Autodesk Fusion 360 part; units mm, degrees
(part 3 of 13)
  line L1812 (141.624, -72.5436) -> (141.627, -72.5391)
  line L1813 (141.22, -72.9625) -> (141.287, -72.9157)
  line L1814 (144.496, -71.2807) -> (144.455, -71.3702)
  line L1815 (141.745, -81.2151) -> (141.668, -81.0591)
  line L1816 (100.087, -70.3919) -> (100.08, -70.4118)
  line L1817 (99.926, -70.1408) -> (99.9333, -70.1465)
  line L1818 (100.059, -70.284) -> (100.065, -70.3008)
  line L1819 (99.9486, -70.1553) -> (99.9571, -70.1588)
  line L1820 (100.08, -70.3362) -> (100.087, -70.3561)
  line L1821 (88.7182, -70.3919) -> (88.7208, -70.374)
  line L1822 (99.8082, -70.6072) -> (99.801, -70.6015)
  line L1823 (99.9871, -70.1888) -> (100.059, -70.284)
  line L1824 (88.8796, -70.1408) -> (88.9008, -70.1378)
  line L1825 (99.9049, -70.6102) -> (99.8851, -70.6182)
  line L1826 (88.8571, -70.5927) -> (88.8485, -70.5892)
  line L1827 (100.085, -70.374) -> (100.087, -70.3919)
  line L1828 (88.8185, -70.1888) -> (88.8353, -70.1756)
  line L1829 (100.087, -70.3561) -> (100.085, -70.374)
  line L1830 (99.9871, -70.5592) -> (99.9703, -70.5724)
  line L1831 (88.7404, -70.4472) -> (88.7292, -70.4329)
  line L1832 (88.9474, -70.6169) -> (88.9385, -70.6192)
  line L1833 (88.9008, -70.6102) -> (88.8796, -70.6072)
  line L1834 (99.8851, -70.6182) -> (99.876, -70.6169)
  line L1835 (88.9297, -70.1311) -> (88.9385, -70.1288)
  line L1836 (100.059, -70.464) -> (99.9871, -70.5592)
  line L1837 (99.9571, -70.1588) -> (99.9703, -70.1756)
  line L1838 (88.7471, -70.464) -> (88.7404, -70.4472)
  line L1839 (88.9206, -70.6182) -> (88.9008, -70.6102)
  line L1840 (100.065, -70.4472) -> (100.059, -70.464)
  line L1841 (88.8353, -70.5724) -> (88.8185, -70.5592)
  line L1842 (88.8485, -70.5892) -> (88.8353, -70.5724)
  line L1843 (99.9703, -70.5724) -> (99.9571, -70.5892)
  line L1844 (88.8635, -70.1489) -> (88.8724, -70.1465)
  line L1845 (88.8796, -70.6072) -> (88.8724, -70.6015)
  line L1846 (99.9571, -70.5892) -> (99.9486, -70.5927)
  line L1847 (99.9049, -70.1378) -> (99.926, -70.1408)
  line L1848 (99.9421, -70.1489) -> (99.9486, -70.1553)
  line L1849 (100.08, -70.4118) -> (100.076, -70.4329)
  line L1850 (99.9333, -70.1465) -> (99.9421, -70.1489)
  line L1851 (88.9385, -70.1288) -> (88.9474, -70.1311)
  line L1852 (99.926, -70.6072) -> (99.9049, -70.6102)
  line L1853 (99.7921, -70.5991) -> (99.7856, -70.5927)
  line L1854 (88.8635, -70.5991) -> (88.8571, -70.5927)
  line L1855 (99.9486, -70.5927) -> (99.9421, -70.5991)
  line L1856 (99.8583, -70.6169) -> (99.8492, -70.6182)
  line L1857 (88.9297, -70.6169) -> (88.9206, -70.6182)
  line L1858 (88.7471, -70.284) -> (88.8185, -70.1888)
  line L1859 (99.6547, -70.3362) -> (99.6577, -70.3151)
  line L1860 (100.065, -70.3008) -> (100.076, -70.3151)
  line L1861 (99.9703, -70.1756) -> (99.9871, -70.1888)
  line L1862 (88.9385, -70.6192) -> (88.9297, -70.6169)
  line L1863 (88.8571, -70.1553) -> (88.8635, -70.1489)
  line L1864 (88.8353, -70.1756) -> (88.8485, -70.1588)
  line L1865 (88.8485, -70.1588) -> (88.8571, -70.1553)
  line L1866 (99.9421, -70.5991) -> (99.9333, -70.6015)
  line L1867 (88.9206, -70.1298) -> (88.9297, -70.1311)
  line L1868 (88.7404, -70.3008) -> (88.7471, -70.284)
  line L1869 (88.8724, -70.1465) -> (88.8796, -70.1408)
  line L1870 (88.7261, -70.3362) -> (88.7292, -70.3151)
  line L1871 (100.076, -70.3151) -> (100.08, -70.3362)
  line L1872 (88.7292, -70.3151) -> (88.7404, -70.3008)
  line L1873 (88.9008, -70.1378) -> (88.9206, -70.1298)
  line L1874 (99.8851, -70.1298) -> (99.9049, -70.1378)
  line L1875 (88.8724, -70.6015) -> (88.8635, -70.5991)
  line L1876 (99.9333, -70.6015) -> (99.926, -70.6072)
  line L1877 (100.076, -70.4329) -> (100.065, -70.4472)
  line L1878 (99.876, -70.1311) -> (99.8851, -70.1298)
  line L1879 (147.689, -96.129) -> (147.754, -96.0856)
  line L1880 (99.7771, -70.5892) -> (99.7639, -70.5724)
  line L1881 (99.6493, -70.374) -> (99.6468, -70.3561)
  line L1882 (99.6757, -70.284) -> (99.7471, -70.1888)
  line L1883 (99.7639, -70.5724) -> (99.7471, -70.5592)
  line L1884 (147.53, -95.6243) -> (147.397, -95.7052)
  line L1885 (99.8082, -70.1408) -> (99.8293, -70.1378)
  line L1886 (146.874, -95.6199) -> (146.867, -95.6177)
  line L1887 (99.7856, -70.1553) -> (99.7921, -70.1489)
  line L1888 (147.754, -96.0856) -> (147.776, -96.0811)
  line L1889 (99.8492, -70.6182) -> (99.8293, -70.6102)
  line L1890 (147.77, -95.5641) -> (147.766, -95.5631)
  line L1891 (147.689, -96.9618) -> (147.645, -96.8969)
  line L1892 (146.8, -95.5969) -> (146.71, -95.5686)
  line L1893 (99.6468, -70.3919) -> (99.6493, -70.374)
  line L1894 (99.8671, -70.1288) -> (99.876, -70.1311)
  line L1895 (147.772, -95.5653) -> (147.77, -95.5641)
  line L1896 (99.7471, -70.5592) -> (99.6757, -70.464)
  line L1897 (147.544, -95.6181) -> (147.53, -95.6243)
  line L1898 (99.7639, -70.1756) -> (99.7771, -70.1588)
  line L1899 (99.7771, -70.1588) -> (99.7856, -70.1553)
  line L1900 (99.8293, -70.1378) -> (99.8492, -70.1298)
  line L1901 (147.645, -96.1939) -> (147.689, -96.129)
  line L1902 (147.63, -96.2704) -> (147.645, -96.1939)
  line L1903 (146.867, -95.6177) -> (146.8, -95.5969)
  line L1904 (147.021, -95.7088) -> (146.874, -95.6199)
  line L1905 (147.385, -95.7145) -> (147.295, -95.8046)
  line L1906 (144.778, -95.5619) -> (144.522, -95.5619)
  line L1907 (99.6757, -70.464) -> (99.6689, -70.4472)
  line L1908 (99.6468, -70.3561) -> (99.6547, -70.3362)
  line L1909 (146.867, -95.6177) -> (146.867, -95.6177)
  line L1910 (147.295, -95.8046) -> (147.232, -95.8387)
  line L1911 (99.8293, -70.6102) -> (99.8082, -70.6072)
  line L1912 (99.7471, -70.1888) -> (99.7639, -70.1756)
  line L1913 (99.6689, -70.3008) -> (99.6757, -70.284)
  line L1914 (99.8671, -70.6192) -> (99.8583, -70.6169)
  line L1915 (99.6689, -70.4472) -> (99.6577, -70.4329)
  line L1916 (147.397, -95.7052) -> (147.385, -95.7145)
  line L1917 (99.801, -70.1465) -> (99.8082, -70.1408)
  line L1918 (99.7921, -70.1489) -> (99.801, -70.1465)
  line L1919 (146.637, -95.5619) -> (146.634, -95.5619)
  line L1920 (99.801, -70.6015) -> (99.7921, -70.5991)
  line L1921 (147.707, -95.5685) -> (147.694, -95.5711)
  line L1922 (99.8583, -70.1311) -> (99.8671, -70.1288)
  line L1923 (147.776, -96.0811) -> (147.776, -95.5805)
  line L1924 (147.754, -97.0052) -> (147.689, -96.9618)
  line L1925 (147.645, -96.8969) -> (147.63, -96.8204)
  line L1926 (99.876, -70.6169) -> (99.8671, -70.6192)
  line L1927 (147.776, -95.5805) -> (147.772, -95.5653)
  line L1928 (147.232, -95.8387) -> (147.162, -95.8336)
  line L1929 (99.8492, -70.1298) -> (99.8583, -70.1311)
  line L1930 (99.6577, -70.3151) -> (99.6689, -70.3008)
  line L1931 (147.116, -95.8046) -> (147.021, -95.7088)
  line L1932 (147.63, -96.8204) -> (147.63, -96.2704)
  line L1933 (147.162, -95.8336) -> (147.116, -95.8046)
  line L1934 (145.036, -95.5619) -> (145.033, -95.5619)
  line L1935 (144.522, -95.5619) -> (144.52, -95.5622)
  line L1936 (99.6577, -70.4329) -> (99.6547, -70.4118)
  line L1937 (147.694, -95.5711) -> (147.544, -95.6181)
  line L1938 (147.766, -95.5631) -> (147.707, -95.5685)
  line L1939 (146.71, -95.5686) -> (146.637, -95.5619)
  line L1940 (145.033, -95.5619) -> (144.778, -95.5619)
  line L1941 (99.7856, -70.5927) -> (99.7771, -70.5892)
  line L1942 (99.6547, -70.4118) -> (99.6468, -70.3919)
  line L1943 (145.265, -95.6177) -> (145.265, -95.6177)
  line L1944 (145.199, -95.5969) -> (145.109, -95.5686)
  line L1945 (146.121, -95.5622) -> (146.121, -95.5622)
  line L1946 (143.762, -93.8918) -> (143.762, -93.8639)
  line L1947 (145.74, -95.7088) -> (145.669, -95.7799)
  line L1948 (145.606, -95.8139) -> (145.536, -95.8088)
  line L1949 (145.887, -95.6199) -> (145.74, -95.7088)
  line L1950 (143.762, -93.9826) -> (143.763, -93.9714)
  line L1951 (143.745, -93.7376) -> (143.745, -93.7376)
  line L1952 (144.293, -95.6177) -> (144.285, -95.6199)
  line L1953 (143.762, -93.86) -> (143.761, -93.8481)
  line L1954 (143.981, -95.8383) -> (143.91, -95.8332)
  line L1955 (145.894, -95.6177) -> (145.894, -95.6177)
  line L1956 (146.044, -95.5706) -> (146.044, -95.5706)
  line L1957 (145.536, -95.8088) -> (145.491, -95.7799)
  line L1958 (146.124, -95.5619) -> (146.121, -95.5622)
  line L1959 (143.762, -93.8639) -> (143.762, -93.86)
  line L1960 (144.519, -95.5622) -> (144.486, -95.5653)
  line L1961 (143.75, -93.7638) -> (143.747, -93.745)
  line L1962 (143.757, -93.795) -> (143.754, -93.7845)
  line L1963 (143.91, -95.8332) -> (143.865, -95.8043)
  line L1964 (145.109, -95.5686) -> (145.036, -95.5619)
  line L1965 (143.76, -93.8118) -> (143.76, -93.8039)
  line L1966 (143.765, -95.6765) -> (143.762, -95.6497)
  line L1967 (143.763, -93.9714) -> (143.765, -93.9639)
  line L1968 (146.044, -95.5706) -> (145.894, -95.6177)
  line L1969 (145.419, -95.7088) -> (145.273, -95.6199)
  line L1970 (146.05, -95.5686) -> (146.044, -95.5706)
  line L1971 (143.747, -93.745) -> (143.745, -93.7376)
  line L1972 (146.087, -95.5653) -> (146.05, -95.5686)
  line L1973 (145.894, -95.6177) -> (145.887, -95.6199)
  line L1974 (145.265, -95.6177) -> (145.199, -95.5969)
  line L1975 (146.121, -95.5622) -> (146.087, -95.5653)
  line L1976 (145.491, -95.7799) -> (145.419, -95.7088)
  line L1977 (144.139, -95.7088) -> (144.043, -95.8043)
  line L1978 (144.043, -95.8043) -> (143.981, -95.8383)
  line L1979 (143.745, -93.7376) -> (143.731, -93.7039)
  line L1980 (143.765, -93.9639) -> (143.763, -93.8958)
  line L1981 (143.76, -93.8039) -> (143.757, -93.795)
  line L1982 (143.799, -95.7388) -> (143.765, -95.6765)
  line L1983 (143.762, -95.6497) -> (143.762, -93.9826)
  line L1984 (143.717, -93.6578) -> (143.717, -93.6578)
  line L1985 (145.273, -95.6199) -> (145.265, -95.6177)
  line L1986 (144.486, -95.5653) -> (144.449, -95.5686)
  line L1987 (146.38, -95.5619) -> (146.124, -95.5619)
  line L1988 (144.52, -95.5622) -> (144.519, -95.5622)
  line L1989 (143.763, -93.8958) -> (143.762, -93.8918)
  line L1990 (143.75, -93.7651) -> (143.75, -93.7638)
  line L1991 (144.443, -95.5706) -> (144.293, -95.6177)
  line L1992 (143.865, -95.8043) -> (143.799, -95.7388)
  line L1993 (143.727, -93.6927) -> (143.717, -93.6578)
  line L1994 (143.754, -93.7845) -> (143.75, -93.7651)
  line L1995 (144.449, -95.5686) -> (144.443, -95.5706)
  line L1996 (145.669, -95.7799) -> (145.606, -95.8139)
  line L1997 (146.634, -95.5619) -> (146.38, -95.5619)
  line L1998 (144.285, -95.6199) -> (144.139, -95.7088)
  line L1999 (144.443, -95.5706) -> (144.443, -95.5706)
  line L2000 (143.731, -93.7039) -> (143.727, -93.6927)
  line L2001 (145.48, -82.2318) -> (145.48, -82.2318)
  line L2002 (143.634, -93.5124) -> (143.619, -93.4981)
  line L2003 (145.955, -82.3539) -> (145.955, -82.3539)
  line L2004 (143.638, -93.5193) -> (143.634, -93.5124)
  line L2005 (145.963, -82.3547) -> (145.963, -82.3547)
  line L2006 (146.164, -82.3559) -> (146.166, -82.3557)
  line L2007 (146.346, -82.3413) -> (146.351, -82.3409)
  line L2008 (145.988, -82.3558) -> (145.989, -82.3559)
  line L2009 (145.815, -82.3297) -> (145.955, -82.3539)
  line L2010 (143.588, -93.4616) -> (143.56, -93.4385)
  line L2011 (144.293, -95.6177) -> (144.293, -95.6177)
  line L2012 (142.604, -92.4116) -> (142.615, -92.3365)
  line L2013 (145.059, -81.9624) -> (145.059, -81.9624)
  line L2014 (143.717, -93.6578) -> (143.715, -93.6502)
  line L2015 (146.166, -82.3557) -> (146.346, -82.3413)
  line L2016 (145.48, -82.2318) -> (145.705, -82.3096)
  line L2017 (143.552, -93.4305) -> (142.987, -92.8662)
  line L2018 (142.617, -92.2782) -> (142.604, -92.136)
  line L2019 (143.656, -93.5505) -> (143.638, -93.5193)
  line L2020 (143.715, -93.6502) -> (143.705, -93.6328)
  line L2021 (143.689, -93.5962) -> (143.663, -93.5604)
  line L2022 (143.761, -93.8481) -> (143.76, -93.8118)
  line L2023 (142.606, -92.4564) -> (142.604, -92.4116)
  line L2024 (143.594, -93.4667) -> (143.588, -93.4616)
  line L2025 (142.987, -92.8662) -> (142.64, -92.5187)
  line L2026 (142.599, -92.0811) -> (142.599, -92.0811)
  line L2027 (143.663, -93.5604) -> (143.656, -93.5505)
  line L2028 (145.258, -82.1141) -> (145.258, -82.1141)
  line L2029 (145.059, -81.9624) -> (145.25, -82.1086)
  line L2030 (145.705, -82.3096) -> (145.712, -82.3118)
  line L2031 (143.599, -93.4731) -> (143.594, -93.4667)
  line L2032 (143.56, -93.4385) -> (143.552, -93.4305)
  line L2033 (145.285, -82.1286) -> (145.475, -82.2302)
  line L2034 (145.989, -82.3559) -> (146.164, -82.3559)
  line L2035 (145.25, -82.1086) -> (145.254, -82.1117)
  line L2036 (145.475, -82.2302) -> (145.48, -82.2318)
  line L2037 (145.959, -82.3545) -> (145.963, -82.3547)
  line L2038 (142.604, -92.136) -> (142.599, -92.0811)
  line L2039 (142.64, -92.5187) -> (142.606, -92.4564)
  line L2040 (143.619, -93.4981) -> (143.606, -93.4831)
  line L2041 (143.588, -93.4616) -> (143.588, -93.4616)
  line L2042 (143.705, -93.6328) -> (143.696, -93.615)
  line L2043 (146.166, -82.3557) -> (146.166, -82.3557)
  line L2044 (145.258, -82.1141) -> (145.285, -82.1286)
  line L2045 (146.589, -82.2822) -> (146.594, -82.281)
  line L2046 (143.696, -93.615) -> (143.691, -93.6036)
  line L2047 (142.615, -92.3365) -> (142.617, -92.2782)
  line L2048 (146.356, -82.3397) -> (146.589, -82.2822)
  line L2049 (143.606, -93.4831) -> (143.599, -93.4731)
  line L2050 (145.712, -82.3118) -> (145.815, -82.3297)
  line L2051 (145.055, -81.9594) -> (145.059, -81.9624)
  line L2052 (143.691, -93.6036) -> (143.689, -93.5962)
  line L2053 (146.356, -82.3397) -> (146.356, -82.3397)
  line L2054 (147.385, -81.6898) -> (147.511, -81.473)
  line L2055 (147.663, -80.7428) -> (147.635, -80.4937)
  line L2056 (146.494, -79.2846) -> (146.49, -79.283)
  line L2057 (146.246, -72.9976) -> (146.28, -72.9625)
  line L2058 (145.25, -82.1086) -> (145.25, -82.1086)
  line L2059 (147.457, -80.0209) -> (147.333, -79.8377)
  line L2060 (147.511, -81.473) -> (147.526, -81.4327)
  line L2061 (147.226, -81.8835) -> (147.385, -81.6898)
  line L2062 (145.254, -82.1117) -> (145.258, -82.1141)
  line L2063 (147.625, -80.4586) -> (147.568, -80.2573)
  line L2064 (147.651, -80.9983) -> (147.652, -80.9934)
  line L2065 (146.821, -82.185) -> (146.825, -82.183)
  line L2066 (147.462, -80.0297) -> (147.462, -80.0297)
  line L2067 (146.687, -72.5391) -> (146.689, -72.5341)
  line L2068 (146.347, -72.9157) -> (146.4, -72.8783)
  line L2069 (147.322, -79.8218) -> (147.322, -79.8218)
  line L2070 (147.635, -80.4937) -> (147.625, -80.4586)
  line L2071 (147.566, -80.2524) -> (147.564, -80.2478)
  line L2072 (146.594, -82.281) -> (146.599, -82.2791)
  line L2073 (145.955, -82.3539) -> (145.959, -82.3545)
  line L2074 (146.821, -82.185) -> (146.821, -82.185)
  line L2075 (147.652, -80.9934) -> (147.657, -80.8824)
  line L2076 (147.599, -81.2436) -> (147.601, -81.2389)
  line L2077 (147.564, -80.2478) -> (147.564, -80.2478)
  line L2078 (147.462, -80.0297) -> (147.46, -80.0251)
  line L2079 (147.601, -81.2389) -> (147.607, -81.2096)
  line L2080 (147.657, -80.8824) -> (147.663, -80.7428)
  line L2081 (146.599, -82.2791) -> (146.599, -82.2791)
  line L2082 (147.037, -82.0494) -> (147.226, -81.8835)
  line L2083 (146.346, -82.3413) -> (146.346, -82.3413)
  line L2084 (145.963, -82.3547) -> (145.988, -82.3558)
  line L2085 (147.333, -79.8377) -> (147.322, -79.8218)
  line L2086 (146.599, -82.2791) -> (146.821, -82.185)
  line L2087 (145.988, -82.3558) -> (145.988, -82.3558)
  line L2088 (147.526, -81.4327) -> (147.599, -81.2436)
  line L2089 (147.568, -80.2572) -> (147.566, -80.2524)
  line L2090 (147.568, -80.2573) -> (147.568, -80.2572)
  line L2091 (147.46, -80.0251) -> (147.457, -80.0209)
  line L2092 (147.322, -79.8218) -> (147.319, -79.8177)
  line L2093 (146.825, -82.183) -> (147.037, -82.0494)
  line L2094 (146.4, -72.8783) -> (146.405, -72.8751)
  line L2095 (147.564, -80.2478) -> (147.462, -80.0297)
  line L2096 (147.607, -81.2096) -> (147.651, -80.9983)
  line L2097 (146.4, -72.8783) -> (146.4, -72.8783)
  line L2098 (147.319, -79.8177) -> (147.147, -79.6354)
  line L2099 (146.351, -82.3409) -> (146.356, -82.3397)
  line L2100 (146.405, -72.8751) -> (146.561, -72.7194)
  line L2101 (146.684, -72.5436) -> (146.687, -72.5391)
  line L2102 (146.905, -79.4602) -> (146.731, -79.367)
  line L2103 (146.561, -72.7194) -> (146.59, -72.6768)
  line L2104 (147.111, -79.6076) -> (146.952, -79.4862)
  line L2105 (146.226, -73.0658) -> (146.246, -72.9976)
  line L2106 (146.331, -79.2555) -> (146.267, -79.2242)
  line L2107 (146.485, -79.2821) -> (146.485, -79.2821)
  line L2108 (146.952, -79.4862) -> (146.952, -79.4862)
  line L2109 (146.59, -72.6768) -> (146.684, -72.5436)
  line L2110 (146.684, -72.5436) -> (146.684, -72.5436)
  line L2111 (146.689, -72.5341) -> (146.689, -72.5341)
  line L2112 (146.727, -79.3646) -> (146.722, -79.363)
  line L2113 (146.28, -72.9625) -> (146.347, -72.9157)
  line L2114 (146.722, -79.363) -> (146.494, -79.2846)
  line L2115 (146.722, -79.363) -> (146.722, -79.363)
  line L2116 (146.267, -79.2242) -> (146.23, -79.1634)
  line L2117 (146.226, -79.1314) -> (146.226, -73.0658)
  line L2118 (147.147, -79.6354) -> (147.111, -79.6076)
  line L2119 (146.731, -79.367) -> (146.727, -79.3646)
  line L2120 (146.948, -79.4831) -> (146.905, -79.4602)
  line L2121 (146.49, -79.283) -> (146.485, -79.2821)
  line L2122 (146.952, -79.4862) -> (146.948, -79.4831)
  line L2123 (146.23, -79.1634) -> (146.226, -79.1314)
  line L2124 (146.778, -72.3445) -> (146.78, -72.3395)
  line L2125 (146.689, -72.5341) -> (146.778, -72.3445)
  line L2126 (145.593, -70.6441) -> (145.373, -70.6633)
  line L2127 (146.561, -71.0954) -> (146.405, -70.9397)
  line L2128 (146.687, -71.2757) -> (146.658, -71.2339)
  line L2129 (146.689, -71.2807) -> (146.689, -71.2807)
  line L2130 (146.837, -71.688) -> (146.78, -71.4753)
  line L2131 (145.161, -70.7203) -> (145.067, -70.7638)
  line L2132 (145.067, -70.7638) -> (144.966, -70.811)
  line L2133 (146.856, -71.9074) -> (146.837, -71.688)
  line L2134 (145.373, -70.6633) -> (145.161, -70.7203)
  line L2135 (144.785, -70.9365) -> (144.781, -70.9397)
  line L2136 (144.781, -70.9397) -> (144.625, -71.0954)
  line L2137 (145.812, -70.6633) -> (145.593, -70.6441)
  line L2138 (144.961, -70.8133) -> (144.957, -70.8165)
  line L2139 (146.564, -71.0999) -> (146.561, -71.0954)
  line L2140 (146.405, -70.9397) -> (146.224, -70.8133)
  line L2141 (144.957, -70.8165) -> (144.785, -70.9365)
  line L2142 (144.957, -70.8165) -> (144.957, -70.8165)
  line L2143 (144.625, -71.0954) -> (144.622, -71.0999)
  line L2144 (146.689, -71.2807) -> (146.687, -71.2757)
  line L2145 (146.658, -71.2339) -> (146.564, -71.0999)
  line L2146 (146.837, -72.1268) -> (146.856, -71.9074)
  line L2147 (144.966, -70.811) -> (144.966, -70.811)
  line L2148 (146.731, -71.3702) -> (146.689, -71.2807)
  line L2149 (146.78, -72.3395) -> (146.837, -72.1268)
  line L2150 (146.564, -71.0999) -> (146.564, -71.0999)
  line L2151 (144.966, -70.811) -> (144.961, -70.8133)
  line L2152 (144.785, -70.9365) -> (144.785, -70.9365)
  line L2153 (144.785, -72.8783) -> (144.839, -72.9157)
  line L2154 (146.224, -70.8133) -> (146.025, -70.7203)
  line L2155 (144.785, -72.8783) -> (144.785, -72.8783)
  line L2156 (146.78, -71.4753) -> (146.731, -71.3702)
  line L2157 (146.025, -70.7203) -> (145.812, -70.6633)
  line L2158 (144.595, -72.6768) -> (144.625, -72.7194)
  line L2159 (146.485, -79.2821) -> (146.331, -79.2555)
  line L2160 (149.909, -80.5669) -> (149.743, -80.582)
  line L2161 (148.697, -80.5093) -> (148.707, -80.5177)
  line L2162 (150.385, -80.9281) -> (150.394, -80.9227)
  line L2163 (150.436, -80.8938) -> (150.444, -80.8833)
  line L2164 (149.764, -81.0945) -> (149.972, -81.0763)
  line L2165 (149.08, -80.1512) -> (149.078, -80.1468)
  line L2166 (149.082, -80.8944) -> (149.122, -80.9227)
  line L2167 (149.753, -81.0945) -> (149.764, -81.0945)
  line L2168 (148.668, -80.4681) -> (148.697, -80.5093)
  line L2169 (150.077, -80.51) -> (150.068, -80.5152)
  line L2170 (150.394, -80.9227) -> (150.436, -80.8938)
  line L2171 (149.079, -80.8706) -> (149.073, -80.8824)
  line L2172 (149.073, -80.8824) -> (149.082, -80.8944)
  line L2173 (148.57, -80.2588) -> (148.574, -80.2691)
  line L2174 (149.332, -81.0203) -> (149.534, -81.0744)
  line L2175 (149.534, -81.0744) -> (149.545, -81.0763)
  line L2176 (150.068, -80.5152) -> (149.909, -80.5669)
  line L2177 (148.516, -80.0568) -> (148.57, -80.2588)
  line L2178 (148.721, -80.5107) -> (149.08, -80.1512)
  line L2179 (150.437, -80.8699) -> (150.077, -80.51)
  line L2180 (148.662, -80.4586) -> (148.668, -80.4681)
  line L2181 (149.972, -81.0763) -> (149.983, -81.0744)
  line L2182 (150.185, -81.0203) -> (150.195, -81.0165)
  line L2183 (150.444, -80.8833) -> (150.437, -80.8699)
  line L2184 (150.195, -81.0165) -> (150.385, -80.9281)
  line L2185 (149.577, -80.5599) -> (149.441, -80.5092)
  circle A0 centre (105.131, -90.8304) radius 0.2
  circle A1 centre (95.4532, -98.5774) radius 0.2
  circle A2 centre (149.733, -79.8322) radius 0.2
  line L2186 (149.764, -78.5699) -> (149.753, -78.5699)
  line L2187 (149.545, -78.5881) -> (149.534, -78.59)
  circle A3 centre (100.914, -89.8144) radius 0.2
  line L2188 (149.534, -78.59) -> (149.332, -78.6441)
  circle A4 centre (124.028, -105.486) radius 0.2
  line L2189 (149.073, -78.7811) -> (149.08, -78.7945)
  circle A5 centre (91.2368, -97.3582) radius 0.2
  line L2190 (149.753, -78.5699) -> (149.545, -78.5881)
  circle A6 centre (96.8756, -86.4362) radius 0.2
  circle A7 centre (107.061, -117.678) radius 0.2
  circle A8 centre (118.694, -110.109) radius 0.2
  line L2191 (149.08, -78.7945) -> (149.439, -79.1536)
  line L2192 (149.081, -78.7706) -> (149.073, -78.7811)
  circle A9 centre (146.444, -102.87) radius 0.2
  line L2193 (149.332, -78.6441) -> (149.322, -78.6479)
  circle A10 centre (102.87, -116.281) radius 0.2
  circle A11 centre (91.3739, -95.631) radius 0.2
  circle A12 centre (105.867, -119.151) radius 0.2
  circle A13 centre (91.1352, -91.8464) radius 0.2
  line L2194 (149.122, -78.7417) -> (149.081, -78.7706)
  circle A14 centre (127.82, -93.8319) radius 0.2
  circle A15 centre (91.2368, -94.4372) radius 0.2
  line L2195 (148.496, -79.8377) -> (148.514, -80.046)
  line L2196 (150.435, -78.77) -> (150.394, -78.7417)
  line L2197 (149.93, -79.102) -> (150.077, -79.1545)
  line L2198 (148.516, -79.6076) -> (148.514, -79.6184)
  line L2199 (148.514, -79.6184) -> (148.496, -79.8267)
  circle A16 centre (86.9442, -111.658) radius 0.2
  line L2200 (149.322, -78.6479) -> (149.132, -78.7363)
  line L2201 (150.385, -78.7363) -> (150.195, -78.6479)
  line L2202 (148.708, -79.1466) -> (148.696, -79.1559)
  circle A17 centre (86.8426, -104.191) radius 0.2
  line L2203 (149.132, -78.7363) -> (149.122, -78.7417)
  line L2204 (148.514, -80.046) -> (148.516, -80.0568)
  line L2205 (149.078, -80.1468) -> (149.025, -79.9881)
  line L2206 (148.662, -79.2058) -> (148.574, -79.3953)
  line L2207 (149.012, -101.459) -> (149.012, -101.459)
  line L2208 (149.368, -101.344) -> (149.361, -101.346)
  line L2209 (149.659, -101.366) -> (149.565, -101.346)
  line L2210 (149.363, -98.3228) -> (149.37, -98.3327)
  line L2211 (149.385, -98.3579) -> (149.392, -98.3708)
  line L2212 (149.432, -98.4165) -> (149.438, -98.4216)
  line L2213 (149.311, -98.233) -> (149.315, -98.2398)
  line L2214 (149.466, -98.4447) -> (149.474, -98.4527)
  line L2215 (149.811, -98.8412) -> (149.811, -101.242)
  line L2216 (148.634, -101.873) -> (148.629, -101.881)
  line L2217 (149.006, -101.462) -> (148.852, -101.574)
  line L2218 (149.308, -101.357) -> (149.181, -101.384)
  line L2219 (149.342, -98.2934) -> (149.363, -98.3228)
  line L2220 (149.281, -98.1456) -> (149.295, -98.1793)
  line L2221 (149.37, -98.3327) -> (149.385, -98.3579)
  line L2222 (149.808, -98.8144) -> (149.811, -98.8412)
  line L2223 (149.181, -101.384) -> (149.175, -101.387)
  line L2224 (149.277, -98.1275) -> (149.279, -98.1382)
  line L2225 (149.392, -98.3708) -> (149.407, -98.3851)
  line L2226 (149.272, -98.0987) -> (149.276, -98.1181)
  line L2227 (149.276, -98.1181) -> (149.277, -98.1275)
  line L2228 (148.852, -101.574) -> (148.724, -101.716)
  line L2229 (149.175, -101.387) -> (149.012, -101.459)
  line L2230 (149.012, -101.459) -> (149.006, -101.462)
  line L2231 (148.337, -102.284) -> (148.32, -102.261)
  line L2232 (149.281, -98.1456) -> (149.281, -98.1456)
  line L2233 (149.565, -101.346) -> (149.565, -101.346)
  line L2234 (148.57, -102.063) -> (148.569, -102.07)
  line L2235 (149.407, -98.3851) -> (149.42, -98.4001)
  line L2236 (148.288, -102.206) -> (148.16, -102.064)
  line L2237 (149.42, -98.4001) -> (149.432, -98.4165)
  line L2238 (149.361, -101.346) -> (149.361, -101.346)
  line L2239 (148.569, -102.07) -> (148.569, -102.07)
  line L2240 (149.474, -98.4527) -> (149.774, -98.7521)
  line L2241 (149.337, -98.287) -> (149.342, -98.2934)
  line L2242 (148.569, -102.07) -> (148.554, -102.212)
  line L2243 (149.342, -98.2934) -> (149.342, -98.2934)
  line L2244 (149.811, -101.242) -> (149.791, -101.311)
  line L2245 (148.16, -102.064) -> (148.061, -101.992)
  line L2246 (149.33, -98.2682) -> (149.337, -98.287)
  line L2247 (149.438, -98.4216) -> (149.466, -98.4447)
  line L2248 (149.737, -101.357) -> (149.667, -101.367)
  line L2249 (149.361, -101.346) -> (149.308, -101.357)
  line L2250 (148.629, -101.881) -> (148.57, -102.063)
  line L2251 (148.724, -101.716) -> (148.721, -101.722)
  line L2252 (148.32, -102.261) -> (148.288, -102.206)
  line L2253 (149.774, -98.7521) -> (149.808, -98.8144)
  line L2254 (148.398, -102.32) -> (148.337, -102.284)
  line L2255 (147.837, -101.877) -> (147.831, -101.874)
  line L2256 (148.469, -102.318) -> (148.398, -102.32)
  line L2257 (148.721, -101.722) -> (148.634, -101.873)
  line L2258 (148.554, -102.212) -> (148.527, -102.277)
  line L2259 (149.667, -101.367) -> (149.659, -101.366)
  line L2260 (149.565, -101.346) -> (149.559, -101.344)
  line L2261 (147.26, -101.877) -> (147.26, -101.877)
  line L2262 (148.527, -102.277) -> (148.469, -102.318)
  line L2263 (149.175, -101.387) -> (149.175, -101.387)
  line L2264 (149.559, -101.344) -> (149.368, -101.344)
  line L2265 (148.011, -101.956) -> (148.005, -101.952)
  line L2266 (144.549, -92.6207) -> (144.546, -92.6946)
  line L2267 (144.582, -92.458) -> (144.55, -92.6156)
  line L2268 (144.6, -92.3751) -> (144.6, -92.3751)
  line L2269 (145.164, -91.5596) -> (144.976, -91.7255)
  line L2270 (144.567, -93.1153) -> (144.568, -93.1202)
  line L2271 (144.976, -91.7255) -> (144.817, -91.9192)
  line L2272 (144.817, -91.9192) -> (144.691, -92.136)
  line L2273 (145.607, -91.328) -> (145.603, -91.3299)
  line L2274 (149.441, -80.5092) -> (149.079, -80.8706)
  line L2275 (149.545, -81.0763) -> (149.753, -81.0945)
  line L2276 (149.983, -81.0744) -> (150.185, -81.0203)
  line L2277 (144.538, -92.8662) -> (144.567, -93.1153)
  line L2278 (145.846, -91.2693) -> (145.614, -91.3263)
  line L2279 (144.6, -92.3751) -> (144.582, -92.458)
  line L2280 (145.846, -91.2693) -> (145.846, -91.2693)
  line L2281 (149.743, -80.582) -> (149.577, -80.5599)
  line L2282 (145.851, -91.2681) -> (145.846, -91.2693)
  line L2283 (145.381, -91.424) -> (145.376, -91.426)
  line L2284 (145.376, -91.426) -> (145.164, -91.5596)
  line L2285 (144.55, -92.6156) -> (144.549, -92.6207)
  line L2286 (144.549, -92.6207) -> (144.549, -92.6207)
  line L2287 (145.603, -91.3299) -> (145.381, -91.424)
  line L2288 (149.122, -80.9227) -> (149.132, -80.9281)
  line L2289 (149.322, -81.0165) -> (149.332, -81.0203)
  line L2290 (145.603, -91.3299) -> (145.603, -91.3299)
  line L2291 (144.546, -92.6946) -> (144.538, -92.8662)
  line L2292 (149.132, -80.9281) -> (149.322, -81.0165)
  line L2293 (145.614, -91.3263) -> (145.607, -91.328)
  line L2294 (150.195, -78.6479) -> (150.185, -78.6441)
  line L2295 (149.439, -79.1536) -> (149.439, -79.1536)
  line L2296 (150.185, -78.6441) -> (149.983, -78.59)
  line L2297 (149.983, -78.59) -> (149.972, -78.5881)
  line L2298 (149.972, -78.5881) -> (149.764, -78.5699)
  line L2299 (148.72, -79.153) -> (148.708, -79.1466)
  line L2300 (150.444, -78.782) -> (150.435, -78.77)
  line L2301 (148.57, -79.4056) -> (148.516, -79.6076)
  line L2302 (149.439, -79.1536) -> (149.597, -79.0997)
  line L2303 (148.696, -79.1559) -> (148.668, -79.1963)
  line L2304 (149.081, -79.514) -> (148.72, -79.153)
  line L2305 (148.707, -80.5177) -> (148.721, -80.5107)
  line L2306 (149.597, -79.0997) -> (149.764, -79.0822)
  line L2307 (150.077, -79.1545) -> (150.438, -78.7938)
  line L2308 (149.008, -79.8217) -> (149.029, -79.6558)
  line L2309 (148.574, -80.2691) -> (148.662, -80.4586)
  line L2310 (149.029, -79.6558) -> (149.081, -79.514)
  line L2311 (148.574, -79.3953) -> (148.57, -79.4056)
  line L2312 (150.394, -78.7417) -> (150.385, -78.7363)
  line L2313 (148.496, -79.8267) -> (148.496, -79.8377)
  line L2314 (149.764, -79.0822) -> (149.93, -79.102)
  line L2315 (150.438, -78.7938) -> (150.444, -78.782)
  line L2316 (148.668, -79.1963) -> (148.662, -79.2058)
  line L2317 (149.025, -79.9881) -> (149.008, -79.8217)
  circle A18 centre (102.184, -89.789) radius 0.2
  circle A19 centre (110.388, -112.928) radius 0.2
  circle A20 centre (106.259, -100.878) radius 0.2
  circle A21 centre (145.085, -112.954) radius 0.2
  circle A22 centre (117.424, -136.703) radius 0.2
  circle A23 centre (105.372, -102.044) radius 0.2
  circle A24 centre (105.359, -108.839) radius 0.2
  circle A25 centre (130.759, -113.157) radius 0.2
  circle A26 centre (116.933, -112.486) radius 0.2
  circle A27 centre (136.322, -110.871) radius 0.2
  line L2318 (146.599, -94.2933) -> (146.821, -94.1992)
  line L2319 (147.651, -93.0125) -> (147.652, -93.0076)
  line L2320 (147.662, -92.7483) -> (147.635, -92.5129)
  line L2321 (147.385, -93.704) -> (147.511, -93.4872)
  line L2322 (146.589, -94.2964) -> (146.594, -94.2952)
  line L2323 (147.511, -93.4872) -> (147.519, -93.4667)
  line L2324 (147.658, -92.8662) -> (147.663, -92.757)
  line L2325 (147.037, -94.0636) -> (147.226, -93.8977)
  line L2326 (146.821, -94.1992) -> (146.821, -94.1992)
  line L2327 (147.652, -93.0076) -> (147.652, -93.0012)
  line L2328 (147.635, -92.5129) -> (147.635, -92.5079)
  line L2329 (146.594, -94.2952) -> (146.599, -94.2933)
  line L2330 (147.625, -93.1393) -> (147.651, -93.0125)
  line L2331 (147.143, -91.6466) -> (146.952, -91.5004)
  line L2332 (146.246, -91.2551) -> (146.246, -91.2551)
  line L2333 (147.219, -91.7255) -> (147.151, -91.6533)
  line L2334 (146.722, -91.3772) -> (146.722, -91.3772)
  line L2335 (146.494, -91.2988) -> (146.49, -91.2972)
  line L2336 (147.319, -91.8319) -> (147.219, -91.7255)
  line L2337 (146.243, -91.2545) -> (146.239, -91.2543)
  line L2338 (146.722, -91.3772) -> (146.494, -91.2988)
  line L2339 (146.212, -91.2531) -> (146.038, -91.2531)
  line L2340 (146.239, -91.2543) -> (146.239, -91.2543)
  line L2341 (147.322, -91.836) -> (147.322, -91.836)
  line L2342 (146.239, -91.2543) -> (146.214, -91.2532)
  line L2343 (147.147, -91.6496) -> (147.143, -91.6466)
  line L2344 (146.035, -91.2533) -> (146.035, -91.2533)
  line L2345 (147.462, -92.0439) -> (147.46, -92.0393)
  line L2346 (147.151, -91.6533) -> (147.147, -91.6496)
  line L2347 (146.214, -91.2532) -> (146.214, -91.2532)
  line L2348 (147.46, -92.0393) -> (147.457, -92.0351)
  line L2349 (146.952, -91.5004) -> (146.948, -91.4973)
  line L2350 (146.214, -91.2532) -> (146.212, -91.2531)
  line L2351 (146.952, -91.5004) -> (146.952, -91.5004)
  line L2352 (146.246, -91.2551) -> (146.243, -91.2545)
  line L2353 (147.322, -91.836) -> (147.319, -91.8319)
  line L2354 (146.49, -91.2972) -> (146.386, -91.2793)
  line L2355 (146.038, -91.2531) -> (146.035, -91.2533)
  line L2356 (146.948, -91.4973) -> (146.727, -91.3788)
  line L2357 (147.457, -92.0351) -> (147.322, -91.836)
  line L2358 (146.386, -91.2793) -> (146.246, -91.2551)
  line L2359 (146.727, -91.3788) -> (146.722, -91.3772)
  line L2360 (145.856, -91.2677) -> (145.856, -91.2677)
  line L2361 (145.856, -91.2677) -> (145.851, -91.2681)
  line L2362 (144.601, -92.3701) -> (144.6, -92.3751)
  line L2363 (144.691, -92.136) -> (144.601, -92.3701)
  line L2364 (146.035, -91.2533) -> (145.856, -91.2677)
  line L2365 (151.744, -97.6456) -> (151.741, -97.638)
  line L2366 (151.786, -97.7917) -> (151.78, -97.7723)
  line L2367 (151.847, -107.016) -> (151.8, -106.962)
  line L2368 (152.598, -72.1999) -> (152.639, -72.2579)
  line L2369 (151.791, -97.9427) -> (151.789, -97.8836)
  line L2370 (152.595, -91.2531) -> (152.553, -106.91)
  line L2371 (151.776, -97.7529) -> (151.776, -97.7516)
  line L2372 (151.791, -97.9517) -> (151.791, -97.9427)
  line L2373 (152.533, -106.978) -> (152.479, -107.024)
  line L2374 (151.771, -97.7254) -> (151.758, -97.6917)
  line L2375 (151.789, -97.9592) -> (151.791, -97.9517)
  line L2376 (152.479, -107.024) -> (152.427, -107.036)
  line L2377 (151.789, -97.8796) -> (151.789, -97.8517)
  line L2378 (151.787, -97.8359) -> (151.786, -97.7996)
  line L2379 (151.754, -97.6805) -> (151.744, -97.6456)
  line L2380 (151.774, -97.7328) -> (151.771, -97.7254)
  line L2381 (151.789, -97.9704) -> (151.789, -97.9592)
  line L2382 (152.646, -72.299) -> (152.595, -91.2531)
  line L2383 (151.789, -97.8836) -> (151.789, -97.8796)
  line L2384 (152.532, -72.1733) -> (152.598, -72.1999)
  line L2385 (152.553, -106.91) -> (152.533, -106.978)
  line L2386 (151.78, -97.7723) -> (151.776, -97.7529)
  line L2387 (151.786, -97.7996) -> (151.786, -97.7917)
  line L2388 (151.8, -106.962) -> (151.789, -106.91)
  line L2389 (151.776, -97.7516) -> (151.774, -97.7328)
  line L2390 (152.639, -72.2579) -> (152.646, -72.299)
  line L2391 (151.915, -107.036) -> (151.847, -107.016)
  line L2392 (151.789, -106.91) -> (151.789, -97.9704)
  line L2393 (151.758, -97.6917) -> (151.754, -97.6805)
  line L2394 (151.741, -97.638) -> (151.731, -97.6206)
  line L2395 (149.667, -70.7539) -> (149.667, -70.7539)
  line L2396 (149.645, -70.811) -> (149.579, -70.9833)
  line L2397 (151.014, -69.8665) -> (150.834, -69.8809)
  line L2398 (150.581, -69.9431) -> (150.46, -69.9944)
  line L2399 (152.197, -70.3387) -> (152.129, -70.2665)
  line L2400 (150.581, -69.9431) -> (150.581, -69.9431)
  line L2401 (149.579, -70.9833) -> (149.528, -71.2288)
  line L2402 (150.834, -69.8809) -> (150.834, -69.8809)
  line L2403 (150.593, -69.9395) -> (150.586, -69.9412)
  line L2404 (150.824, -69.8825) -> (150.593, -69.9395)
  line L2405 (150.834, -69.8809) -> (150.829, -69.8813)
  line L2406 (151.217, -69.8675) -> (151.192, -69.8664)
  line L2407 (151.365, -69.8925) -> (151.225, -69.8683)
  line L2408 (151.7, -69.9904) -> (151.7, -69.9904)
  line L2409 (151.225, -69.8683) -> (151.221, -69.8677)
  line L2410 (151.217, -69.8675) -> (151.217, -69.8675)
  line L2411 (150.355, -70.0392) -> (150.143, -70.1728)
  line L2412 (152.125, -70.2628) -> (152.121, -70.2598)
  line L2413 (150.46, -69.9944) -> (150.355, -70.0392)
  line L2414 (152.576, -70.6691) -> (152.506, -70.679)
  line L2415 (151.926, -70.1105) -> (151.705, -69.992)
  line L2416 (149.795, -70.5324) -> (149.669, -70.7492)
  line L2417 (151.191, -69.8663) -> (151.016, -69.8663)
  line L2418 (135.399, -70.6306) -> (135.348, -70.5812)
  line L2419 (149.669, -70.7492) -> (149.667, -70.7539)
  line L2420 (150.824, -69.8825) -> (150.824, -69.8825)
  line L2421 (151.192, -69.8664) -> (151.192, -69.8664)
  line L2422 (150.829, -69.8813) -> (150.824, -69.8825)
  line L2423 (151.221, -69.8677) -> (151.217, -69.8675)
  line L2424 (135.331, -70.519) -> (135.331, -69.4417)
  line L2425 (151.016, -69.8663) -> (151.014, -69.8665)
  line L2426 (150.143, -70.1728) -> (149.954, -70.3387)
  line L2427 (152.654, -69.3169) -> (152.65, -70.5546)
  line L2428 (151.014, -69.8665) -> (151.014, -69.8665)
  line L2429 (151.192, -69.8664) -> (151.191, -69.8663)
  line L2430 (151.473, -69.912) -> (151.468, -69.9104)
  line L2431 (150.586, -69.9412) -> (150.581, -69.9431)
  line L2432 (152.65, -70.5546) -> (152.63, -70.6227)
  line L2433 (149.954, -70.3387) -> (149.795, -70.5324)
  line L2434 (151.225, -69.8683) -> (151.225, -69.8683)
  line L2435 (152.298, -70.4451) -> (152.197, -70.3387)
  line L2436 (152.301, -70.4493) -> (152.301, -70.4493)
  line L2437 (149.667, -70.7539) -> (149.645, -70.811)
  line L2438 (151.468, -69.9104) -> (151.365, -69.8925)
  line L2439 (151.705, -69.992) -> (151.7, -69.9904)
  line L2440 (151.334, -72.9671) -> (151.568, -72.9096)
  line L2441 (149.547, -71.7334) -> (149.547, -71.7334)
  line L2442 (152.204, -72.5109) -> (152.363, -72.3172)
  line L2443 (149.616, -71.9744) -> (149.616, -71.9744)
  line L2444 (150.232, -72.7391) -> (150.453, -72.8576)
  line L2445 (151.324, -72.9687) -> (151.324, -72.9687)
  line L2446 (149.614, -71.9698) -> (149.616, -71.9744)
  line L2447 (150.037, -72.5898) -> (150.228, -72.736)
  line L2448 (149.545, -71.7285) -> (149.547, -71.7334)
  line L2449 (152.462, -72.1865) -> (152.532, -72.1733)
  line L2450 (149.616, -71.9744) -> (149.718, -72.1925)
  line L2451 (150.037, -72.5898) -> (150.037, -72.5898)
  line L2452 (150.941, -72.9821) -> (150.966, -72.9832)
  line L2453 (149.547, -71.7334) -> (149.596, -71.9074)
  line L2454 (149.723, -72.2013) -> (149.858, -72.4004)
  line L2455 (149.596, -71.9074) -> (149.614, -71.9698)
  line L2456 (150.684, -72.937) -> (150.69, -72.9392)
  line L2457 (149.526, -71.2807) -> (149.517, -71.4794)
  line L2458 (151.334, -72.9671) -> (151.334, -72.9671)
  line L2459 (150.794, -72.9571) -> (150.934, -72.9813)
  line L2460 (151.799, -72.8124) -> (151.804, -72.8104)
  line L2461 (151.142, -72.9833) -> (151.145, -72.9831)
  line L2462 (149.964, -72.5143) -> (150.033, -72.5868)
  line L2463 (149.528, -71.2339) -> (149.526, -71.2807)
  line L2464 (149.861, -72.4045) -> (149.864, -72.4082)
  line L2465 (151.577, -72.9065) -> (151.577, -72.9065)
  line L2466 (150.458, -72.8592) -> (150.684, -72.937)
  line L2467 (150.453, -72.8576) -> (150.458, -72.8592)
  line L2468 (150.458, -72.8592) -> (150.458, -72.8592)
  line L2469 (149.72, -72.1971) -> (149.723, -72.2013)
  line L2470 (149.517, -71.4794) -> (149.545, -71.7285)
  line L2471 (150.966, -72.9832) -> (150.968, -72.9833)
  line L2472 (149.723, -72.2013) -> (149.723, -72.2013)
  line L2473 (149.858, -72.4004) -> (149.861, -72.4045)
  line L2474 (151.577, -72.9065) -> (151.799, -72.8124)
  line L2475 (149.718, -72.1925) -> (149.72, -72.1971)
  line L2476 (152.366, -72.3128) -> (152.411, -72.2353)
  line L2477 (150.228, -72.736) -> (150.232, -72.7391)
  line L2478 (149.864, -72.4082) -> (149.964, -72.5143)
  line L2479 (149.858, -72.4004) -> (149.858, -72.4004)
  line L2480 (151.568, -72.9096) -> (151.573, -72.9084)
  line L2481 (152.366, -72.3128) -> (152.366, -72.3128)
  line L2482 (150.033, -72.5868) -> (150.037, -72.5898)
  line L2483 (149.864, -72.4082) -> (149.864, -72.4082)
  line L2484 (150.228, -72.736) -> (150.228, -72.736)
  line L2485 (152.363, -72.3172) -> (152.366, -72.3128)
  line L2486 (152.411, -72.2353) -> (152.462, -72.1865)
  line L2487 (150.934, -72.9813) -> (150.934, -72.9813)
  line L2488 (149.528, -71.2288) -> (149.528, -71.2339)
  line L2489 (149.528, -71.2339) -> (149.528, -71.2339)
  line L2490 (151.799, -72.8124) -> (151.799, -72.8124)
  line L2491 (151.324, -72.9687) -> (151.329, -72.9683)
  line L2492 (150.941, -72.9821) -> (150.941, -72.9821)
  line L2493 (151.145, -72.9831) -> (151.145, -72.9831)
  line L2494 (151.329, -72.9683) -> (151.334, -72.9671)
  line L2495 (152.016, -72.6768) -> (152.204, -72.5109)
  line L2496 (150.934, -72.9813) -> (150.937, -72.9819)
  line L2497 (150.966, -72.9832) -> (150.966, -72.9832)
  line L2498 (151.145, -72.9831) -> (151.324, -72.9687)
  line L2499 (151.804, -72.8104) -> (152.016, -72.6768)
  line L2500 (150.968, -72.9833) -> (151.142, -72.9833)
  line L2501 (150.937, -72.9819) -> (150.941, -72.9821)
  line L2502 (151.573, -72.9084) -> (151.577, -72.9065)
  line L2503 (151.771, -97.7254) -> (151.771, -97.7254)
  line L2504 (152.427, -107.036) -> (151.915, -107.036)
  line L2505 (151.789, -97.8517) -> (151.788, -97.8478)
  line L2506 (151.788, -97.8478) -> (151.787, -97.8359)
  line L2507 (150.69, -72.9392) -> (150.794, -72.9571)
  line L2508 (147.568, -92.2715) -> (147.568, -92.2715)
  line L2509 (147.226, -93.8977) -> (147.385, -93.704)
  line L2510 (146.599, -94.2933) -> (146.599, -94.2933)
  line L2511 (147.568, -92.2715) -> (147.566, -92.2666)
  line L2512 (146.356, -94.3539) -> (146.356, -94.3539)
  line L2513 (147.566, -92.2666) -> (147.564, -92.262)
  line L2514 (146.821, -94.1992) -> (146.825, -94.1972)
  line L2515 (147.564, -92.262) -> (147.564, -92.262)
  line L2516 (147.519, -93.4667) -> (147.569, -93.3347)
  line L2517 (147.652, -93.0012) -> (147.658, -92.8662)
  line L2518 (147.663, -92.757) -> (147.662, -92.7483)
  line L2519 (146.825, -94.1972) -> (147.037, -94.0636)
  line L2520 (147.601, -93.2531) -> (147.625, -93.1393)
  line L2521 (146.356, -94.3539) -> (146.589, -94.2964)
  line L2522 (147.564, -92.262) -> (147.462, -92.0439)
  line L2523 (147.462, -92.0439) -> (147.462, -92.0439)
  line L2524 (147.569, -93.3347) -> (147.601, -93.2531)
  line L2525 (144.886, -93.795) -> (144.886, -93.795)
  line L2526 (145.955, -94.3681) -> (145.959, -94.3687)
  line L2527 (145.48, -94.246) -> (145.705, -94.3238)
  line L2528 (145.254, -94.1259) -> (145.258, -94.1283)
  line L2529 (145.963, -94.3689) -> (145.963, -94.3689)
  line L2530 (145.705, -94.3238) -> (145.712, -94.326)
  line L2531 (145.059, -93.9766) -> (145.059, -93.9766)
  line L2532 (145.959, -94.3687) -> (145.963, -94.3689)
  line L2533 (144.886, -93.795) -> (144.986, -93.9011)
  line L2534 (145.055, -93.9736) -> (145.059, -93.9766)
  line L2535 (145.059, -93.9766) -> (145.25, -94.1228)
  line L2536 (145.258, -94.1283) -> (145.258, -94.1283)
  line L2537 (145.988, -94.37) -> (145.989, -94.3701)
  line L2538 (147.596, -92.3701) -> (147.568, -92.2715)
  line L2539 (145.48, -94.246) -> (145.48, -94.246)
  line L2540 (145.963, -94.3689) -> (145.988, -94.37)
  line L2541 (145.955, -94.3681) -> (145.955, -94.3681)
  line L2542 (145.989, -94.3701) -> (146.164, -94.3701)
  line L2543 (146.164, -94.3701) -> (146.166, -94.3699)
  line L2544 (144.986, -93.9011) -> (145.055, -93.9736)
  line L2545 (145.25, -94.1228) -> (145.254, -94.1259)
  line L2546 (145.258, -94.1283) -> (145.329, -94.1662)
  line L2547 (147.635, -92.5079) -> (147.596, -92.3701)
  line L2548 (146.353, -97.9768) -> (146.355, -97.9571)
  line L2549 (146.127, -98.409) -> (146.173, -98.3593)
  line L2550 (146.342, -98.0399) -> (146.351, -98.0047)
  line L2551 (146.33, -98.1024) -> (146.333, -98.0951)
  line L2552 (145.476, -99.0569) -> (145.781, -98.7521)
  line L2553 (146.34, -98.0515) -> (146.342, -98.0399)
  line L2554 (146.355, -97.9571) -> (146.357, -97.9449)
  line L2555 (146.269, -98.242) -> (146.273, -98.2348)
  line L2556 (146.333, -98.0951) -> (146.334, -98.0873)
  line L2557 (145.442, -106.659) -> (145.444, -106.651)
  line L2558 (145.411, -106.828) -> (145.415, -106.816)
  line L2559 (146.319, -98.1324) -> (146.325, -98.1137)
  line L2560 (146.246, -98.2746) -> (146.257, -98.258)
  line L2561 (146.24, -98.2854) -> (146.24, -98.2854)
  line L2562 (145.444, -102.352) -> (145.439, -102.324)
  line L2563 (145.444, -103.4) -> (145.444, -102.352)
  line L2564 (145.439, -106.595) -> (145.439, -103.416)
  line L2565 (146.357, -97.9449) -> (146.358, -97.9371)
  line L2566 (146.236, -98.2923) -> (146.24, -98.2854)
  line L2567 (146.351, -98.0047) -> (146.351, -98.0047)
  line L2568 (145.399, -106.866) -> (145.401, -106.858)
  line L2569 (145.428, -106.754) -> (145.437, -106.719)
  line L2570 (146.33, -98.1024) -> (146.33, -98.1024)
  line L2571 (145.439, -106.711) -> (145.439, -106.691)
  line L2572 (145.439, -106.691) -> (145.44, -106.671)
  line L2573 (145.401, -106.858) -> (145.401, -106.858)
  line L2574 (145.444, -106.651) -> (145.439, -106.607)
  line L2575 (145.459, -99.0779) -> (145.476, -99.0569)
  line L2576 (145.781, -98.7521) -> (146.112, -98.4206)
  line L2577 (145.44, -106.671) -> (145.442, -106.659)
  line L2578 (145.439, -106.607) -> (145.439, -106.595)
  line L2579 (146.24, -98.2854) -> (146.246, -98.2746)
  line L2580 (146.273, -98.2348) -> (146.287, -98.2015)
  line L2581 (146.257, -98.258) -> (146.257, -98.2576)
  line L2582 (146.287, -98.2015) -> (146.292, -98.1908)
  line L2583 (145.437, -106.719) -> (145.437, -106.719)
  line L2584 (146.313, -98.1521) -> (146.319, -98.1324)
  line L2585 (146.176, -98.3565) -> (146.196, -98.3368)
  line L2586 (146.12, -98.4131) -> (146.127, -98.409)
  line L2587 (145.437, -106.719) -> (145.439, -106.711)
  line L2588 (145.439, -103.416) -> (145.444, -103.4)
  line L2589 (145.392, -106.892) -> (145.398, -106.868)
  line L2590 (146.207, -98.3235) -> (146.236, -98.2923)
  line L2591 (146.325, -98.1137) -> (146.33, -98.1024)
  line L2592 (146.273, -98.2348) -> (146.273, -98.2348)
  line L2593 (146.257, -98.2576) -> (146.269, -98.242)
  line L2594 (146.334, -98.0873) -> (146.334, -98.0873)
  line L2595 (145.439, -102.324) -> (145.439, -99.146)
  line L2596 (146.206, -98.3246) -> (146.207, -98.3235)
  line L2597 (145.439, -99.146) -> (145.459, -99.0779)
  line L2598 (146.112, -98.4206) -> (146.12, -98.4131)
  line L2599 (146.353, -97.997) -> (146.353, -97.9768)
  line L2600 (146.354, -97.893) -> (146.353, -97.8812)
  line L2601 (146.351, -98.0047) -> (146.353, -97.997)
  line L2602 (147.295, -97.2862) -> (147.385, -97.3763)
  line L2603 (146.373, -97.5868) -> (146.427, -97.5403)
  line L2604 (146.64, -97.5286) -> (146.675, -97.5254)
  line L2605 (146.874, -97.4709) -> (147.021, -97.382)
  line L2606 (147.775, -97.5225) -> (147.776, -97.5149)
  line L2607 (146.63, -97.5289) -> (146.637, -97.5289)
  line L2608 (147.707, -97.5223) -> (147.762, -97.5273)
  line L2609 (148.367, -97.5197) -> (148.516, -97.4727)
  line L2610 (146.358, -97.9371) -> (146.354, -97.893)
  line L2611 (150.508, -79.8322) -> (150.508, -79.8531)
  line L2612 (148.66, -97.3516) -> (148.571, -97.2631)
  line L2613 (148.571, -97.2631) -> (148.514, -97.1516)
  line L2614 (147.25, -97.2572) -> (147.295, -97.2862)
  line L2615 (146.718, -97.5197) -> (146.867, -97.4731)
  line L2616 (148.372, -96.9618) -> (148.307, -97.0052)
  line L2617 (148.676, -97.3763) -> (148.687, -97.3653)
  line L2618 (148.514, -96.9044) -> (148.541, -96.8514)
  line L2619 (147.116, -97.2862) -> (147.179, -97.2521)
  line L2620 (146.71, -97.5222) -> (146.718, -97.5197)
  line L2621 (146.637, -97.5289) -> (146.64, -97.5286)
  line L2622 (148.294, -97.5277) -> (148.354, -97.5223)
  line L2623 (148.687, -97.3653) -> (148.66, -97.3516)
  line L2624 (147.776, -97.0097) -> (147.754, -97.0052)
  line L2625 (148.489, -96.7994) -> (148.43, -96.7994)
  line L2626 (146.479, -97.5289) -> (146.63, -97.5289)
  line L2627 (146.334, -98.0873) -> (146.34, -98.0515)
  line L2628 (146.353, -97.6549) -> (146.373, -97.5868)
  line L2629 (146.867, -97.4731) -> (146.874, -97.4709)
  line L2630 (148.53, -97.4665) -> (148.664, -97.3856)
  line L2631 (147.773, -97.5239) -> (147.775, -97.5225)
  line L2632 (146.292, -98.1908) -> (146.313, -98.1521)
  line L2633 (147.694, -97.5197) -> (147.707, -97.5223)
  line L2634 (147.397, -97.3856) -> (147.53, -97.4665)
  line L2635 (146.64, -97.5286) -> (146.64, -97.5286)
  line L2636 (147.179, -97.2521) -> (147.25, -97.2572)
  line L2637 (147.544, -97.4727) -> (147.694, -97.5197)
  line L2638 (147.762, -97.5273) -> (147.773, -97.5239)
  line L2639 (146.675, -97.5254) -> (146.71, -97.5222)
  line L2640 (146.353, -97.8812) -> (146.353, -97.6549)
  line L2641 (147.776, -97.5149) -> (147.776, -97.0097)
  line L2642 (148.29, -97.5267) -> (148.294, -97.5277)
  line L2643 (148.495, -97.028) -> (148.514, -96.9044)
  line L2644 (147.385, -97.3763) -> (147.397, -97.3856)
  line L2645 (148.664, -97.3856) -> (148.676, -97.3763)
  line L2646 (146.427, -97.5403) -> (146.479, -97.5289)
  line L2647 (147.53, -97.4665) -> (147.544, -97.4727)
  line L2648 (148.516, -97.4727) -> (148.53, -97.4665)
  line L2649 (148.415, -96.8969) -> (148.372, -96.9618)
  line L2650 (148.284, -97.0097) -> (148.284, -97.5103)
  line L2651 (148.541, -96.8514) -> (148.489, -96.7994)
  line L2652 (148.514, -97.1516) -> (148.495, -97.028)
  line L2653 (146.198, -98.3336) -> (146.206, -98.3246)
  line L2654 (150.49, -79.666) -> (150.508, -79.8322)
  line L2655 (148.354, -97.5223) -> (148.367, -97.5197)
  line L2656 (148.289, -97.5255) -> (148.29, -97.5267)
  line L2657 (147.021, -97.382) -> (147.116, -97.2862)
  line L2658 (146.196, -98.3368) -> (146.198, -98.3336)
  line L2659 (146.867, -97.4731) -> (146.867, -97.4731)
  line L2660 (147.831, -107.036) -> (145.516, -107.036)
  line L2661 (146.494, -103.815) -> (147.92, -105.241)
  line L2662 (145.988, -103.661) -> (145.994, -103.664)
  line L2663 (146.633, -101.981) -> (146.546, -101.963)
  line L2664 (147.266, -101.874) -> (147.26, -101.877)
  line L2665 (147.098, -101.949) -> (147.092, -101.952)
  line L2666 (147.092, -101.952) -> (147.087, -101.956)
  line L2667 (147.447, -101.836) -> (147.447, -101.836)
  line L2668 (147.087, -101.956) -> (147.087, -101.956)
  line L2669 (147.087, -101.956) -> (146.97, -102.041)
  line L2670 (148.061, -101.992) -> (148.011, -101.956)
  line L2671 (147.737, -101.854) -> (147.651, -101.836)
  line L2672 (146.97, -102.041) -> (146.903, -102.064)
  line L2673 (147.26, -101.877) -> (147.098, -101.949)
  line L2674 (147.999, -101.949) -> (147.837, -101.877)
  line L2675 (147.831, -101.874) -> (147.737, -101.854)
  line L2676 (146.845, -102.054) -> (146.733, -102.004)
  line L2677 (147.837, -101.877) -> (147.837, -101.877)
  line L2678 (147.92, -105.241) -> (147.954, -105.304)
  line L2679 (147.954, -105.304) -> (147.957, -105.33)
  line L2680 (147.957, -105.33) -> (147.957, -106.91)
  line L2681 (146.903, -102.064) -> (146.845, -102.054)
  line L2682 (147.883, -107.024) -> (147.831, -107.036)
  line L2683 (146.349, -101.962) -> (146.342, -101.963)